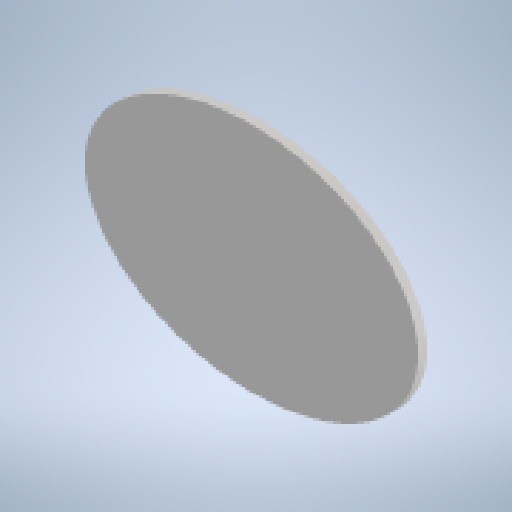
# Autodesk Inventor part: Деталь1
Saved by Autodesk Inventor 2023.1 (Build 271208000, 208)
## iProperties
Created: 2024-11-15
Part Number: Деталь1
Material: Типовые
Document SubType Name: Modeling
Designer: DELL
Density: 1 g/cm^3
Appearance: По умолчанию
Author: DELL
Autodesk Inventor part; units mm, degrees
ref_plane "YZ Plane" through (0, 0, 0) normal (1, 0, 0) x (0, 1, 0)
ref_plane "XZ Plane" through (0, 0, 0) normal (0, 1, 0) x (-1, 0, 0)
ref_plane "XY Plane" through (0, 0, 0) normal (0, 0, 1) x (1, 0, 0)
ref_plane "РабПлоскость1" through (0, 0, 0) normal (0, 0, 1) x (1, 0, 0)
sketch "Эскиз1" plane through (0, 0, 0) normal (0, 0, 1) x (1, 0, 0)
  line L0 (-172.9092, -12.3688) -> (-172.9092, 7.6312) construction
  line L1 (28.5504, 6.1312) -> (-172.9092, -12.3688) construction
  ellipse E0 centre (-72.1794, -3.1188) end of major axis (-192.177, -2.3565) minor radius 79.9991
  point P0 (0, 0)
  point P1 (-72.1794, -83.1188)
  dimension "d2" = 120
  dimension "d3" = 80
  constraints: 2 end point, 1 midpoint, 1 vertical alignment, 3 other
  measures "d3" distance of point (-72.179, -83.119) point (-72.179, -3.119)
extrude "Выдавливание1" add sketch "Эскиз1" along normal blind 6
